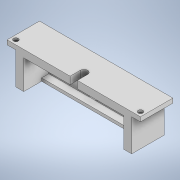
# Autodesk Inventor part: bottomcameraholder_6_24_2021
Saved by Autodesk Inventor 2021 (Build 250183000, 183)
## iProperties
Created: 2021-06-18
Part Number: bottomcameraholder_6_24_2021
Material: Generic
Document SubType Name: Modeling
Designer: erenc
Density: 1 g/cm^3
Appearance: Default
Author: erenc
Autodesk Inventor part; units mm, degrees
ref_plane "YZ Plane" through (0, 0, 0) normal (1, 0, 0) x (0, 1, 0)
ref_plane "XZ Plane" through (0, 0, 0) normal (0, 1, 0) x (-1, 0, 0)
ref_plane "XY Plane" through (0, 0, 0) normal (0, 0, 1) x (1, 0, 0)
sketch "Sketch2" plane through (0, 0, 0) normal (0, 1, 0) x (-1, 0, 0)
  line L0 (0, 0) -> (0, -39.2)
  line L1 (0, -39.2) -> (-69.3, -39.2)
  line L2 (-69.3, -39.2) -> (-69.3, 0)
  line L3 (-69.3, 0) -> (0, 0)
  dimension "d0" = 39.2
  dimension "d1" = 69.3
  constraints: 8 end point, 3 perpendicular, 1 vertical
  measures "d0" distance of L0.start L0.end
  measures "d1" distance of L0.end L1.end
extrude "Extrusion1" add sketch "Sketch2" against normal blind 5
sketch "Sketch3" plane through (0, -5, 0) normal (0, -1, 0) x (1, 0, 0)
  line L0 (0, 0) -> (0, -39.2) projected
  line L1 (0, -39.2) -> (0, -34.2)
  line L2 (0, -34.2) -> (69.3, -34.2)
  line L3 (69.3, -39.2) -> (69.3, 0) projected
  line L4 (69.3, -39.2) -> (69.3, -34.2)
  line L5 (0, -39.2) -> (69.3, -39.2)
  dimension "d4" = 5
  constraints: 8 end point, 3 perpendicular, 2 point on line
  measures "d4" distance of L0.end L1.end
extrude "Extrusion2" add sketch "Sketch3" along normal blind 20
sketch "Sketch4" plane through (0, -5, -34.2) normal (0, 0, 1) x (1, 0, 0)
  line L0 (0, 5) -> (0, -20) projected
  line L1 (0, -20) -> (0, -18)
  line L2 (0, -18) -> (69.3, -18)
  line L3 (69.3, 5) -> (69.3, -20) projected
  line L4 (69.3, -20) -> (69.3, -18)
  line L5 (0, -20) -> (69.3, -20) projected
  line L6 (0, -20) -> (69.3, -20)
  dimension "d7" = 2
  constraints: 8 end point, 2 point on line, 1 collinear, 1 horizontal, 1 perpendicular
  measures "d7" distance of L0.end L1.end
extrude "Extrusion3" add sketch "Sketch4" along normal blind 5
sketch "Sketch5" plane through (69.3, 0, 0) normal (1, 0, 0) x (0, 0, -1)
  line L0 (39.2, -25) -> (29.2, -25) projected
  line L1 (29.2, -25) -> (29.2, 0)
  line L2 (39.2, 0) -> (0, 0) projected
  line L3 (29.2, 0) -> (39.2, 0)
  line L4 (39.2, 0) -> (39.2, -25)
  line L5 (39.2, -25) -> (29.2, -25)
  constraints: 8 end point, 2 perpendicular, 1 collinear, 1 vertical
extrude "Extrusion4" add sketch "Sketch5" along normal blind 5
sketch "Sketch6" plane through (69.3, -5, 0) normal (1, 0, 0) x (0, 0, -1)
  line L0 (0, 5) -> (0, 0) projected
  line L1 (29.2, 0) -> (29.2, 5) projected
  line L2 (0, 5) -> (29.2, 5)
  line L3 (29.2, 5) -> (29.2, 0)
  line L4 (0, 0) -> (34.2, 0) projected
  line L5 (29.2, 0) -> (0, 0)
  line L6 (0, 0) -> (0, 5)
  constraints: 8 end point, 2 perpendicular, 1 collinear, 1 horizontal
extrude "Extrusion5" add sketch "Sketch6" along normal blind 5
sketch "Sketch7" plane through (0, -5, -29.2) normal (0, 0, 1) x (1, 0, 0)
  line L0 (0, -20) -> (74.3, -20) projected
  line L1 (74.3, -20) -> (74.3, 0)
  line L2 (74.3, 0) -> (69.3, 0) projected
  line L3 (74.3, 0) -> (69.3, 0)
  line L4 (69.3, 0) -> (69.3, -18) projected
  line L5 (69.3, 0) -> (69.3, -20)
  line L6 (74.3, -20) -> (69.3, -20)
  point P0 (0, 5)
  constraints: 8 end point, 3 perpendicular, 1 point on line
extrude "Extrusion6" add sketch "Sketch7" along normal up to surface (29.2 mm away)
sketch "Sketch8" plane through (0, 0, -39.2) normal (-1, 0, 0) x (0, 0, 1)
  line L0 (10, -25) -> (39.2, -25) projected
  line L1 (10, -25) -> (10, 0)
  line L2 (0, 0) -> (39.2, 0) projected
  line L3 (0, 0) -> (10, 0)
  line L4 (0, 0) -> (0, -25)
  line L5 (0, -25) -> (10, -25)
  constraints: 8 end point, 2 perpendicular, 2 vertical, 1 point on line
extrude "Extrusion7" add sketch "Sketch8" along normal blind 5
sketch "Sketch9" plane through (0, -5, 0) normal (-1, 0, 0) x (0, 0, 1)
  line L0 (-29.2, 5) -> (0, 5) projected
  line L1 (0, 5) -> (-29.2, 5)
  line L2 (-39.2, -20) -> (-29.2, -20) projected
  line L3 (-29.2, 5) -> (-29.2, -20)
  line L4 (0, 5) -> (0, -20) projected
  line L5 (-29.2, -20) -> (0, -20)
  line L6 (0, -20) -> (0, 5)
  constraints: 8 end point, 2 perpendicular, 1 collinear, 1 horizontal
extrude "Extrusion8" add sketch "Sketch9" along normal blind 5
sketch "Sketch10" plane through (74.3, 0, 0) normal (1, 0, 0) x (0, 0, -1)
  line L0 (0, 0) -> (0, -25) projected
  line L1 (0, 0) -> (0, -3)
  line L2 (0, -3) -> (39.2, -3)
  line L3 (39.2, 0) -> (39.2, -25) projected
  line L4 (39.2, 0) -> (0, 0) projected
  line L5 (39.2, 0) -> (0, 0)
  line L6 (39.2, -3) -> (39.2, 0)
  dimension "d20" = 3
  constraints: 8 end point, 2 point on line, 1 horizontal, 1 perpendicular, 1 vertical
  measures "d20" distance of L0.start L1.end
sketch "Sketch11" plane through (-5, 0, -39.2) normal (-1, 0, 0) x (0, 0, 1)
  line L0 (39.2, 0) -> (39.2, -25) projected
  line L1 (39.2, 0) -> (39.2, -3)
  line L2 (39.2, -3) -> (0, -3)
  line L3 (0, 0) -> (0, -25) projected
  line L4 (0, 0) -> (0, -3)
  line L5 (0, 0) -> (39.2, 0)
  dimension "d21" = 3
  constraints: 8 end point, 3 perpendicular, 2 point on line
  measures "d21" distance of L0.start L1.end
extrude "Extrusion9" add sketch "Sketch11" along normal blind 6
extrude "Extrusion10" add sketch "Sketch10" along normal blind 6
sketch "Sketch13" plane through (0, -5, 0) normal (0, -1, 0) x (1, 0, 0)
  line L0 (0, -34.2) -> (69.3, -34.2) projected
  arc A0 (32.15, -24) -> (37.15, -24) centre (34.65, -24) ccw
  line L1 (32.15, -24) -> (32.15, 0)
  line L2 (37.15, -24) -> (37.15, 0)
  line L3 (0, 0) -> (69.3, 0) projected
  dimension "d34" = 5
  dimension "d56" = 24
  dimension "d57" = 24
  constraints: 4 end point, 2 point on circle, 2 vertical, 1 centre point, 1 point on line
  measures "d34" diameter of A0
  measures "d56" distance of L2.start L2.end
  measures "d57" distance of L1.start L1.end
extrude "Extrusion13" cut sketch "Sketch13" against normal through all
sketch "Sketch15" plane through (0, 0, -39.2) normal (1, 0, 0) x (0, 0, -1)
  line L0 (0, -25) -> (-39.2, -25) projected
  line L1 (-10, -23) -> (-10, -25) projected
  line L2 (-39.2, -25) -> (-10, -25)
  line L3 (-10, -25) -> (-10, -23)
  line L4 (-5, -5) -> (-5, -23) projected
  line L5 (-10, -23) -> (-5, -23)
  line L6 (-5, -23) -> (-5, -5)
  line L7 (-39.2, -5) -> (-5, -5) projected
  line L8 (-5, -5) -> (-39.2, -5)
  line L9 (-10, -25) -> (-39.2, -25) projected
  line L10 (-39.2, -5) -> (-39.2, -25)
  point P0 (-39.2, 0)
  constraints: 12 end point, 5 perpendicular, 1 collinear
extrude "Extrusion15" add sketch "Sketch15" along normal blind 0.4
sketch "Sketch16" plane through (69.3, 0, 0) normal (-1, 0, 0) x (0, 0, 1)
  line L0 (-34.2, -5) -> (0, -5) projected
  line L1 (0, -5) -> (0, -25)
  line L2 (-29.2, -25) -> (-29.2, -23) projected
  line L3 (0, -25) -> (-29.2, -25)
  line L4 (-29.2, -25) -> (-29.2, -23)
  line L5 (-29.2, -23) -> (-34.2, -23)
  line L6 (-34.2, -5) -> (-34.2, -23) projected
  line L7 (-34.2, -23) -> (-34.2, -5)
  line L8 (-34.2, -5) -> (0, -5)
  point P0 (0, 0)
  constraints: 12 end point, 5 perpendicular
extrude "Extrusion16" add sketch "Sketch16" along normal blind 0.4
sketch "Sketch17" plane through (0.4, -23, -34.2) normal (0, 0, 1) x (1, 0, 0)
  line L0 (0, 0) -> (30, 0)
  line L1 (0, 0) -> (68.5, 0) projected
  line L2 (68.5, 0) -> (37.5, 0)
  line L3 (37.5, 0) -> (37.5, 3)
  line L4 (30, 0) -> (30, 3)
  line L5 (30, 3) -> (30.8, 3)
  line L6 (37.5, 3) -> (36.7, 3)
  line L7 (34.3, 8.5) -> (30.8, 8.5)
  line L8 (30.8, 8.5) -> (30.8, 3)
  line L9 (36.7, 3) -> (30.8, 3)
  arc A0 (34.3, 3) -> (34.3, 8.5) centre (34.3, 5.75) ccw
  point P0 (-0.4, 23)
  dimension "d46" = 30
  dimension "d47" = 31
  dimension "d48" = 3
  dimension "d49" = 0.8
  dimension "d50" = 0.8
  dimension "d59" = 3.5
  dimension "d60" = 3.5
  dimension "d61" = 5.5
  constraints: 18 end point, 3 horizontal, 2 perpendicular, 2 point on circle, 2 point on line, 2 vertical, 1 centre point, 1 tangent
  measures "d46" distance of L0.start L0.end
  measures "d47" distance of L1.end L2.end
  measures "d48" distance of L2.end L3.end
  measures "d49" distance of L4.end L5.end
  measures "d50" distance of L3.end L6.end
  measures "d59" distance of L7.start L7.end
  measures "d60" distance of A0.start L5.end
  measures "d61" distance of L7.end L5.end
extrude "Extrusion17" add sketch "Sketch17" along normal blind 3 contours L8 L7 A0 L9
sketch "Sketch18" plane through (-11, -3, 0) normal (0, 0, 1) x (1, 0, 0)
  line L0 (6, 0) -> (0, 0) projected
  line L1 (0, 3) -> (0, 0)
  line L2 (0, 0) -> (6, 0)
  line L3 (6, 0) -> (6, -22) projected
  line L4 (6, 0) -> (6, -22)
  line L5 (6, -22) -> (11, -22)
  line L6 (85.3, -22) -> (6, -22) projected
  line L7 (11.4, -2) -> (11.4, -22) projected
  line L8 (11.4, -2) -> (79.9, -2)
  line L9 (79.9, -20) -> (11.4, -20) projected
  line L10 (79.9, -2) -> (79.9, -22)
  line L11 (85.3, -22) -> (85.3, 0) projected
  line L12 (79.9, -22) -> (85.3, -22)
  line L13 (85.3, -22) -> (85.3, 0)
  line L14 (85.3, 0) -> (91.3, 0)
  line L15 (91.3, 0) -> (93.4951, 0)
  line L16 (85.3, 0) -> (91.3, 0) projected
  line L17 (91.3, 0) -> (91.3, 3)
  line L18 (91.3, 3) -> (0, 3)
  line L19 (11.4, -2) -> (79.9, -2) projected
  line L20 (11.4, -2) -> (11.4, -22)
  line L21 (11, -22) -> (11.4, -22)
  point P0 (11, 3)
  constraints: 28 end point, 7 perpendicular, 3 point on line, 3 vertical, 1 horizontal, 1 parallel
extrude "Extrusion18" cut sketch "Sketch18" against normal blind 17 contours L0 L1 L18 L17 L14 L11 L6 L10 L8 L7 L5 L3
sketch "Sketch19" plane through (-11, -3, -39.2) normal (0, -1, 0) x (1, 0, 0)
  line L0 (0, 22.2) -> (0, 0) projected
  line L1 (0, 11.1) -> (6, 11.1)
  line L2 (6, 0) -> (6, 22.2) projected
  circle A0 centre (3, 3) radius 1.65 projected
  circle A1 centre (3, 3) radius 1.65
  circle A2 centre (3, 3) radius 2.5
  circle A3 centre (3, 19.2) radius 1.65
  circle A4 centre (3, 19.2) radius 2.5
  circle A5 centre (88.3, 3) radius 1.65 projected
  circle A6 centre (88.3, 3) radius 1.65
  circle A7 centre (88.3, 3) radius 2.5
  circle A8 centre (88.3, 19.2) radius 1.65
  circle A9 centre (88.3, 19.2) radius 2.5
  point P0 (11, 39.2)
  dimension "d64" = 5
  dimension "d65" = 5
  constraints: 8 centre point, 5 coincident, 4 symmetric about line, 2 end point, 2 midpoint, 4 other
  measures "d64" diameter of A2
  measures "d65" diameter of A7
extrude "Extrusion19" cut sketch "Sketch19" against normal through all contours A3 | A8
extrude "Extrusion20" cut sketch "Sketch19" against normal blind 1.5 contours A3 | A4 | A9
body "Solid1"
